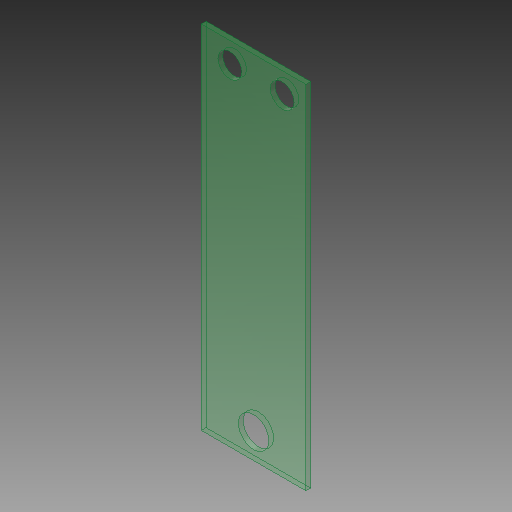
# Autodesk Inventor part: tank_back_2
Saved by Autodesk Inventor 2018.1 (Build 221171000, 171)
## iProperties
Created: 2017-07-30
Part Number: tank_back_2
Material: PVC-Piping
Document SubType Name: Modeling
Designer: Tom
Density: 1.4 g/cm^3
Appearance: Clear - Green 1
Mass: 213.774 g
Surface Area: 812.025 cm^2
Volume: 152.696 cm^3
Author: Tom
Autodesk Inventor part; units mm, degrees
ref_plane "YZ Plane" through (0, 0, 0) normal (1, 0, 0) x (0, 1, 0)
ref_plane "XZ Plane" through (0, 0, 0) normal (0, 1, 0) x (-1, 0, 0)
ref_plane "XY Plane" through (0, 0, 0) normal (0, 0, 1) x (1, 0, 0)
sketch "Sketch1" plane through (0, 0, 0) normal (0, 0, 1) x (1, 0, 0)
  line L0 (0, 0) -> (110, 0)
  line L1 (110, 0) -> (110, 370)
  line L2 (110, 370) -> (0, 370)
  line L3 (0, 370) -> (0, 0)
  dimension "d0" = 110
  dimension "d1" = 370
  constraints: 8 end point, 2 parallel, 1 horizontal, 1 perpendicular
  measures "d0" distance of L2.end L1.end
  measures "d1" distance of L1.end L0.end
extrude "Extrusion1" add sketch "Sketch1" along normal blind 5
sketch "Sketch2" plane through (0, 0, 5) normal (0, 0, 1) x (1, 0, 0)
  line L0 (110, 370) -> (0, 370) construction
  line L1 (55, 370) -> (55, 0) construction
  line L2 (0, 0) -> (110, 0) construction
  circle A0 centre (55, 26) radius 16
  circle A1 centre (30, 347.5) radius 12.5
  circle A2 centre (85, 347.5) radius 12.5
  dimension "d4" = 32
  dimension "d7" = 26
  dimension "d13" = 25
  dimension "d14" = 25
  dimension "d15" = 55
  dimension "d16" = 50
  dimension "d17" = 22.5
  constraints: 3 centre point, 2 end point, 2 midpoint, 1 point on line
  measures "d4" diameter of A0
  measures "d7" distance from line of L2 A0.centre
  measures "d13" diameter of A1
  measures "d14" diameter of A2
  measures "d15" distance of A2.centre A1.centre
  measures "d16" diameter of A1.centre L1
  measures "d17" distance from line of L0 A1.centre
extrude "Extrusion2" cut sketch "Sketch2" against normal blind 5
equation "\"d0\" = tankw + 2 * pvct"
equation "\"d1\" = tankh"
equation "\"d2\" = pvct"
equation "\"d4\" = diaair"
equation "\"d7\" = holeh"
equation "\"d13\" = diawater"
equation "\"d14\" = diaoverflow"
equation "\"d15\" = mindist - 0.5 * diawater - 0.5 * diaoverflow"
equation "\"d16\" = diawater + diaoverflow"
equation "\"d17\" = distfromedge + 0.5 * diawater"
equation "\"d10\" = pvct"
equation "\"lcsd\" = 19.05"
equation "\"lcwd1\" = 25"
equation "\"lcwd2\" = 34"
equation "\"lch1\" = 39"
equation "\"lcwd3\" = 43"
equation "\"dia1\" = 6"
equation "\"td\" = 18"
equation "\"bhh\" = 6"
equation "\"sw\" = 25"
equation "\"sh\" = 31"
equation "\"spacert\" = 2"
equation "\"pvct\" = 5"
equation "\"tankh\" = 370"
equation "\"tankl\" = 379"
equation "\"dia3\" = 8"
equation "\"dia4\" = 11"
equation "\"play\" = 9"
equation "\"holeh\" = 26"
equation "\"surroundt\" = 5"
equation "\"slack\" = 0.5"
equation "\"play2\" = 3"
equation "\"diawater\" = 25"
equation "\"diaph\" = 32"
equation "\"diaair\" = 32"
equation "\"diaoverflow\" = 25"
equation "\"diacucl\" = 32"
equation "\"diasurroundhole\" = 42"
equation "\"diagrate\" = 12"
equation "\"gratespacing\" = 12.02082"
equation "\"bottomdist\" = 9.6355"
equation "\"sidedist\" = 13.9375"
equation "\"diahcl\" = 32"
equation "\"bracketwtop\" = 6"
equation "\"bracketwbottom\" = 6"
equation "\"nett\" = 1"
equation "\"nethole\" = 16"
equation "\"netside\" = 3.5"
equation "\"nettop\" = 7"
equation "\"netholespacing\" = 2"
equation "\"diaetape\" = 32"
equation "\"tankw\" = 100"
equation "\"mindist\" = 80"
equation "\"distfromedge\" = 10"
body "Solid1"
